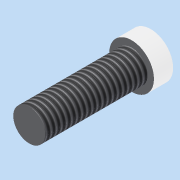
# Autodesk Inventor part: m5x16m
Saved by Autodesk Inventor 2015 (Build 190159000, 159)
## iProperties
Created: 2016-09-08
Part Number: m5x16m
Material: Generic
Document SubType Name: Modeling
Designer: Dustin
Density: 1 g/cm^3
Appearance: Default
Author: Dustin
Autodesk Inventor part; units mm, degrees
ref_plane "YZ Plane" through (0, 0, 0) normal (1, 0, 0) x (0, 1, 0)
ref_plane "XZ Plane" through (0, 0, 0) normal (0, 1, 0) x (-1, 0, 0)
ref_plane "XY Plane" through (0, 0, 0) normal (0, 0, 1) x (1, 0, 0)
sketch "Sketch1" plane through (0, 0, 0) normal (1, 0, 0) x (0, 1, 0)
  line L0 (0, 0) -> (16, 0)
  line L1 (16, 0) -> (16, -2.5)
  line L2 (16, -2.5) -> (0, -2.5)
  line L3 (0, -2.5) -> (0, 0)
  line L4 (16, 0) -> (19, 0)
  line L5 (19, 0) -> (19, -3.5)
  line L6 (19, -3.5) -> (16, -3.5)
  line L7 (16, -3.5) -> (16, 0)
  dimension "d0" = 2.5
  dimension "d1" = 3
  dimension "d2" = 3.5
  dimension "d3" = 16
  constraints: 16 end point, 4 parallel, 2 horizontal, 2 perpendicular
  measures "d0" distance of L2.end L0.start
  measures "d1" distance of L5.end L6.end
  measures "d2" distance of L4.end L5.end
  measures "d3" distance of L0.start L0.end
revolve "Revolution1" add sketch "Sketch1" angle 360 about axis through (0, 0, 0) along (0, 1, 0)
thread "Thread1" size "M5x0.8" class "6g" standard "ANSI Metric M Profile" full length
sketch "Sketch2" plane through (0, 19, 0) normal (0, 1, 0) x (1, 0, 0)
  circle A0 centre (0, 0) radius 2.5 projected
  line L0 (0, 2.5) -> (2.1651, 1.25)
  line L1 (2.1651, 1.25) -> (2.1651, -1.25)
  line L2 (2.1651, -1.25) -> (0, -2.5)
  line L3 (0, -2.5) -> (-2.1651, -1.25)
  line L4 (-2.1651, -1.25) -> (-2.1651, 1.25)
  line L5 (-2.1651, 1.25) -> (0, 2.5)
  constraints: 12 end point, 1 coincident, 1 vertical alignment, 14 other
extrude "Extrusion1" cut sketch "Sketch2" against normal blind 2 contours L1 L2 L3 L4 L5 L0
body "Solid1"
